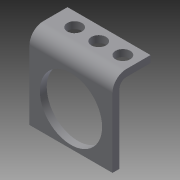
# Autodesk Inventor part: Bearing Mount 2 v1
Saved by Autodesk Inventor 2013 (Build 170138000, 138)
## iProperties
Created: 2013-01-17
Part Number: Bearing Mount 2 v1
Material: Generic
Document SubType Name: Sheet Metal
Designer: actoennies
Density: 1 g/cm^3
Sheet Metal Rule: Default
Mass: 5.60414 g
Surface Area: 46.7484 cm^2
Volume: 5.60414 cm^3
Author: actoennies
Autodesk Inventor part; units mm, degrees
ref_plane "YZ Plane" through (0, 0, 0) normal (1, 0, 0) x (0, 1, 0)
ref_plane "XZ Plane" through (0, 0, 0) normal (0, 1, 0) x (-1, 0, 0)
ref_plane "XY Plane" through (0, 0, 0) normal (0, 0, 1) x (1, 0, 0)
sketch "Sketch1" plane through (0, 0, 0) normal (0, 1, 0) x (-1, 0, 0)
  line L0 (0, 0) -> (34.8343, 0)
  line L1 (34.8343, 0) -> (34.8343, 31.75)
  line L2 (34.8343, 31.75) -> (0, 31.75)
  line L3 (0, 31.75) -> (0, 0)
  circle A0 centre (6.35, 6.35) radius 3.3782
  circle A1 centre (17.4171, 6.35) radius 3.3782
  circle A2 centre (28.4843, 6.35) radius 3.3782
  dimension "d0" = 34.8343
  dimension "d2" = 31.75
  dimension "d3" = 6.7564
  dimension "d4" = 6.7564
  dimension "d5" = 11.0671
  dimension "d6" = 6.7564
  dimension "d7" = 11.0671
  dimension "d8" = 6.35
  dimension "d9" = 6.35
  dimension "d10" = 6.35
  dimension "d11" = 6.35
  measures "d0" distance of L1.end L2.end
  measures "d2" distance of L0.end L1.end
  measures "d3" diameter of A0
  measures "d4" diameter of A1
  measures "d5" distance of A0.centre A1.centre
  measures "d6" diameter of A2
  measures "d7" distance of A1.centre A2.centre
  measures "d8" distance from line of L3 A0.centre
  measures "d9" distance from line of L0 A0.centre
  measures "d10" distance from line of L0 A1.centre
  measures "d11" distance from line of L0 A2.centre
extrude "Plate1" add sketch "Sketch1" along normal blind 3.175
sketch "Sketch4" plane through (-34.8343, 0, 31.75) normal (0, 0, 1) x (1, 0, 0)
  line L0 (34.8343, 0) -> (0, 0)
  line L1 (0, 0) -> (0, -41.275)
  line L2 (0, -41.275) -> (34.8343, -41.275)
  line L3 (34.8343, -41.275) -> (34.8343, 0)
  constraints: 6 end point, 1 horizontal, 1 perpendicular, 1 vertical
edge flange "Flange1" height 44.45 angle 90 thickness 3.175 bend radius 3.175 thickness toward (0, 0, 1) relief straight relief width 3.175 relief depth 1.5875 edges at (-17.4171, 0, 31.75) wall of the first edge with corners at (0, 0, 31.75) (-34.8343, 0, 31.75) (-34.8343, -41.275, 31.75) (0, -41.275, 31.75)
bend "Bend2"
corner "Corner1"
sketch "Sketch5" plane through (-34.8343, -41.275, 34.925) normal (0, 0, 1) x (1, 0, 0)
  circle A0 centre (17.4171, 19.05) radius 14.2875
  line L0 (34.8343, 0) -> (0, 0) projected
  line L1 (34.8343, 38.1) -> (0, 38.1) projected
  line L2 (17.4171, 38.1) -> (17.4171, 0) construction
  point P0 (34.8343, 41.275)
  dimension "d38" = 28.575
  dimension "d41" = 19.05
  dimension "d43" = 0
  constraints: 2 end point, 2 midpoint, 1 centre point
  measures "d38" diameter of A0
  measures "d41" distance from line of L0 A0.centre
  measures "d43" distance from line of A0.centre L2
extrude "Cut1" cut sketch "Sketch5" against normal blind 3.175
sketch "Sketch6" plane through (0, -41.275, 31.75) normal (0, 0, -1) x (-1, 0, 0)
  line L0 (0, 0) -> (0, 38.1) projected
  line L1 (0, 0) -> (34.8343, 0) projected
  line L2 (34.8343, 0) -> (34.8343, 38.1) projected
  arc A0 (22.1343, 0) -> (34.8343, 12.7) centre (22.1343, 12.7) ccw
  arc A1 (0, 12.7) -> (12.7, 0) centre (12.7, 12.7) ccw
  point P0 (0, 41.275)
  dimension "d44" = 25.4
  dimension "d47" = 25.4
  constraints: 4 point on circle, 4 point on line, 4 tangent, 2 centre point
  measures "d44" diameter of A0
  measures "d47" diameter of A1
extrude "Cut2" cut sketch "Sketch6" against normal blind 3.175
equation "\"d39\" = Thickness"
equation "\"d48\" = Thickness"
equation "\"d28\" = BendReliefWidth"
equation "\"d29\" = BendReliefDepth"
equation "\"d30\" = MinimumRemnant"
equation "\"d31\" = BendRadius"
equation "\"d34\" = BendRadius"
equation "\"d35\" = CornerReliefSize"
equation "\"d36\" = GapSize"
equation "\"d37\" = JacobiRadiusSize"
equation "\"BendRadius\" = Thickness"
equation "\"BendReliefWidth\" = Thickness"
equation "\"BendReliefDepth\" = 0.5 * Thickness"
equation "\"CornerReliefSize\" = 4 * Thickness"
equation "\"MinimumRemnant\" = 2 * Thickness"
equation "\"TransitionRadius\" = BendRadius"
equation "\"JacobiRadiusSize\" = BendRadius"
equation "\"GapSize\" = Thickness"
equation "\"d12\" = BendRadius"
equation "\"Thickness\" = 3.175"
body "Solid1"
